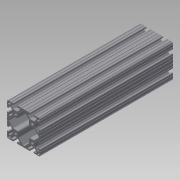
# Autodesk Inventor part: 3030-LITE
Saved by Autodesk Inventor 2013 (Build 170138000, 138)
## iProperties
Created: 2014-04-23
Part Number: 3030-LITE
Material: Generic
Document SubType Name: Modeling
Density: 1 g/cm^3
Vendor: 80/20 Inc.
Engineer: Ross Bowman
Designer: Ross Bowman
Catalog Web Link: 8020.net
Company: 80/20 Inc.
Author: Ross Bowman
Keywords: 80/20 , 8020 , T-Slot , Extrusion
Material: 6105-T5 Aluminum
Autodesk Inventor part; units mm, degrees
ref_plane "YZ Plane" through (0, 0, 0) normal (1, 0, 0) x (0, 1, 0)
ref_plane "XZ Plane" through (0, 0, 0) normal (0, 1, 0) x (-1, 0, 0)
ref_plane "XY Plane" through (0, 0, 0) normal (0, 0, 1) x (1, 0, 0)
sketch "Sketch1" plane through (0, 0, 0) normal (0, 0, 1) x (1, 0, 0)
  circle A0 centre (19.05, -19.05) radius 3.2677
  circle A1 centre (-19.05, -19.05) radius 3.2677
  circle A2 centre (19.05, 19.05) radius 3.2677
  circle A3 centre (-19.05, 19.05) radius 3.2677
  arc A4 (31.2928, -30.9118) -> (30.9118, -31.2928) centre (31.2928, -31.2928) ccw
  line L0 (35.9156, -30.9118) -> (31.2928, -30.9118)
  arc A5 (36.2966, -31.2928) -> (35.9156, -30.9118) centre (35.9156, -31.2928) ccw
  line L1 (36.2966, -33.5026) -> (36.2966, -31.2928)
  arc A6 (33.5026, -36.2966) -> (36.2966, -33.5026) centre (33.5026, -33.5026) ccw
  line L2 (31.2928, -36.2966) -> (33.5026, -36.2966)
  arc A7 (30.9118, -35.9156) -> (31.2928, -36.2966) centre (31.2928, -35.9156) ccw
  line L3 (30.9118, -31.2928) -> (30.9118, -35.9156)
  arc A8 (-35.9156, -30.9118) -> (-36.2966, -31.2928) centre (-35.9156, -31.2928) ccw
  line L4 (-31.2928, -30.9118) -> (-35.9156, -30.9118)
  arc A9 (-30.9118, -31.2928) -> (-31.2928, -30.9118) centre (-31.2928, -31.2928) ccw
  line L5 (-30.9118, -35.9156) -> (-30.9118, -31.2928)
  arc A10 (-31.2928, -36.2966) -> (-30.9118, -35.9156) centre (-31.2928, -35.9156) ccw
  line L6 (-33.5026, -36.2966) -> (-31.2928, -36.2966)
  arc A11 (-36.2966, -33.5026) -> (-33.5026, -36.2966) centre (-33.5026, -33.5026) ccw
  line L7 (-36.2966, -31.2928) -> (-36.2966, -33.5026)
  arc A12 (35.9156, 30.9118) -> (36.2966, 31.2928) centre (35.9156, 31.2928) ccw
  line L8 (31.2928, 30.9118) -> (35.9156, 30.9118)
  arc A13 (30.9118, 31.2928) -> (31.2928, 30.9118) centre (31.2928, 31.2928) ccw
  line L9 (30.9118, 35.9156) -> (30.9118, 31.2928)
  arc A14 (31.2928, 36.2966) -> (30.9118, 35.9156) centre (31.2928, 35.9156) ccw
  line L10 (33.5026, 36.2966) -> (31.2928, 36.2966)
  arc A15 (36.2966, 33.5026) -> (33.5026, 36.2966) centre (33.5026, 33.5026) ccw
  line L11 (36.2966, 31.2928) -> (36.2966, 33.5026)
  arc A16 (-10.9278, 25.0169) -> (-12.319, 21.6583) centre (-7.5692, 21.6583) ccw
  line L12 (-2.0655, 33.8793) -> (-10.9278, 25.0169)
  arc A17 (2.0655, 33.8793) -> (-2.0655, 33.8793) centre (0, 31.8138) ccw
  line L13 (10.9278, 25.0169) -> (2.0655, 33.8793)
  arc A18 (12.319, 21.6583) -> (10.9278, 25.0169) centre (7.5692, 21.6583) ccw
  line L14 (12.319, 15.494) -> (12.319, 21.6583)
  arc A19 (12.319, 15.494) -> (15.494, 12.319) centre (15.494, 15.494) ccw
  line L15 (21.6583, 12.319) -> (15.494, 12.319)
  arc A20 (25.0169, 10.9278) -> (21.6583, 12.319) centre (21.6583, 7.5692) ccw
  line L16 (33.8793, 2.0655) -> (25.0169, 10.9278)
  arc A21 (33.8793, -2.0655) -> (33.8793, 2.0655) centre (31.8138, 0) ccw
  line L17 (25.0169, -10.9278) -> (33.8793, -2.0655)
  arc A22 (21.6583, -12.319) -> (25.0169, -10.9278) centre (21.6583, -7.5692) ccw
  line L18 (15.494, -12.319) -> (21.6583, -12.319)
  arc A23 (15.494, -12.319) -> (12.319, -15.494) centre (15.494, -15.494) ccw
  line L19 (12.319, -21.6583) -> (12.319, -15.494)
  arc A24 (10.9278, -25.0169) -> (12.319, -21.6583) centre (7.5692, -21.6583) ccw
  line L20 (2.0655, -33.8793) -> (10.9278, -25.0169)
  arc A25 (-2.0655, -33.8793) -> (2.0655, -33.8793) centre (0, -31.8138) ccw
  line L21 (-10.9278, -25.0169) -> (-2.0655, -33.8793)
  arc A26 (-12.319, -21.6583) -> (-10.9278, -25.0169) centre (-7.5692, -21.6583) ccw
  line L22 (-12.319, -15.494) -> (-12.319, -21.6583)
  arc A27 (-12.319, -15.494) -> (-15.494, -12.319) centre (-15.494, -15.494) ccw
  line L23 (-21.6583, -12.319) -> (-15.494, -12.319)
  arc A28 (-25.0169, -10.9278) -> (-21.6583, -12.319) centre (-21.6583, -7.5692) ccw
  line L24 (-33.8793, -2.0655) -> (-25.0169, -10.9278)
  arc A29 (-33.8793, 2.0655) -> (-33.8793, -2.0655) centre (-31.8138, 0) ccw
  line L25 (-25.0169, 10.9278) -> (-33.8793, 2.0655)
  arc A30 (-21.6583, 12.319) -> (-25.0169, 10.9278) centre (-21.6583, 7.5692) ccw
  line L26 (-15.494, 12.319) -> (-21.6583, 12.319)
  arc A31 (-15.494, 12.319) -> (-12.319, 15.494) centre (-15.494, 15.494) ccw
  line L27 (-12.319, 21.6583) -> (-12.319, 15.494)
  arc A32 (-31.2928, 30.9118) -> (-30.9118, 31.2928) centre (-31.2928, 31.2928) ccw
  line L28 (-35.9156, 30.9118) -> (-31.2928, 30.9118)
  arc A33 (-36.2966, 31.2928) -> (-35.9156, 30.9118) centre (-35.9156, 31.2928) ccw
  line L29 (-36.2966, 33.5026) -> (-36.2966, 31.2928)
  arc A34 (-33.5026, 36.2966) -> (-36.2966, 33.5026) centre (-33.5026, 33.5026) ccw
  line L30 (-31.2928, 36.2966) -> (-33.5026, 36.2966)
  arc A35 (-30.9118, 35.9156) -> (-31.2928, 36.2966) centre (-31.2928, 35.9156) ccw
  line L31 (-30.9118, 31.2928) -> (-30.9118, 35.9156)
  arc A36 (-3.2004, -38.1) -> (-4.7244, -38.1) centre (-3.9624, -38.1) ccw
  line L32 (-3.2004, -38.1) -> (3.2004, -38.1)
  arc A37 (4.7244, -38.1) -> (3.2004, -38.1) centre (3.9624, -38.1) ccw
  line L33 (4.7244, -38.1) -> (9.5504, -38.1)
  arc A38 (11.0744, -38.1) -> (9.5504, -38.1) centre (10.3124, -38.1) ccw
  line L34 (11.0744, -38.1) -> (13.4107, -38.1)
  arc A39 (13.4107, -38.1) -> (14.986, -36.5252) centre (13.4112, -36.5252) ccw
  line L35 (14.986, -36.5252) -> (14.986, -35.6108)
  arc A40 (14.986, -35.6108) -> (13.4112, -34.036) centre (13.4112, -35.6108) ccw
  line L36 (13.4112, -34.036) -> (12.5733, -34.036)
  arc A41 (12.5733, -34.036) -> (12.192, -34.417) centre (12.573, -34.417) ccw
  line L37 (12.192, -34.417) -> (12.192, -34.4932)
  arc A42 (11.811, -34.8742) -> (12.192, -34.4932) centre (11.811, -34.4932) ccw
  line L38 (11.811, -34.8742) -> (10.033, -34.8742)
  arc A43 (8.763, -33.6042) -> (10.033, -34.8742) centre (10.033, -33.6042) ccw
  line L39 (8.763, -33.6042) -> (8.763, -32.0193)
  arc A44 (9.135, -31.1203) -> (8.763, -32.0193) centre (10.033, -32.0183) ccw
  line L40 (9.135, -31.1203) -> (13.0807, -27.1745)
  arc A45 (16.4417, -25.781) -> (13.0807, -27.1745) centre (16.4417, -30.5308) ccw
  line L41 (16.4417, -25.781) -> (21.6583, -25.781)
  arc A46 (25.0169, -27.1722) -> (21.6583, -25.781) centre (21.6583, -30.5308) ccw
  line L42 (25.0169, -27.1722) -> (28.965, -31.1203)
  arc A47 (29.337, -32.0183) -> (28.965, -31.1203) centre (28.067, -32.0183) ccw
  line L43 (29.337, -32.0183) -> (29.337, -33.6018)
  arc A48 (28.067, -34.8742) -> (29.337, -33.6018) centre (28.067, -33.6042) ccw
  line L44 (28.067, -34.8742) -> (26.289, -34.8742)
  arc A49 (25.908, -34.4932) -> (26.289, -34.8742) centre (26.289, -34.4932) ccw
  line L45 (25.908, -34.4932) -> (25.908, -34.417)
  arc A50 (25.908, -34.417) -> (25.527, -34.036) centre (25.527, -34.417) ccw
  line L46 (25.527, -34.036) -> (24.6894, -34.036)
  arc A51 (24.6894, -34.036) -> (23.114, -35.6108) centre (24.6888, -35.6108) ccw
  line L47 (23.114, -35.6108) -> (23.114, -36.5252)
  arc A52 (23.114, -36.5252) -> (24.6888, -38.1) centre (24.6888, -36.5252) ccw
  line L48 (24.6888, -38.1) -> (27.0256, -38.1)
  arc A53 (28.5496, -38.1) -> (27.0256, -38.1) centre (27.7876, -38.1) ccw
  line L49 (28.5496, -38.1) -> (33.3756, -38.1)
  arc A54 (34.8996, -38.0999) -> (33.3756, -38.1) centre (34.1376, -38.1) ccw
  arc A55 (34.8996, -38.0999) -> (38.0999, -34.8996) centre (34.925, -34.925) ccw
  arc A56 (38.1, -33.3756) -> (38.0999, -34.8996) centre (38.1, -34.1376) ccw
  line L50 (38.1, -33.3756) -> (38.1, -28.5496)
  arc A57 (38.1, -27.0256) -> (38.1, -28.5496) centre (38.1, -27.7876) ccw
  line L51 (38.1, -27.0256) -> (38.1, -24.6893)
  arc A58 (38.1, -24.6893) -> (36.5252, -23.114) centre (36.5252, -24.6888) ccw
  line L52 (36.5252, -23.114) -> (35.6118, -23.114)
  arc A59 (35.6118, -23.114) -> (34.036, -24.6888) centre (35.6108, -24.6888) ccw
  line L53 (34.036, -24.6888) -> (34.036, -25.5253)
  arc A60 (34.036, -25.5253) -> (34.417, -25.908) centre (34.417, -25.527) ccw
  line L54 (34.417, -25.908) -> (34.4929, -25.908)
  arc A61 (34.8742, -26.289) -> (34.4929, -25.908) centre (34.4932, -26.289) ccw
  line L55 (34.8742, -26.289) -> (34.8742, -28.067)
  arc A62 (33.6042, -29.337) -> (34.8742, -28.067) centre (33.6042, -28.067) ccw
  line L56 (33.6042, -29.337) -> (32.0183, -29.337)
  arc A63 (31.1203, -28.965) -> (32.0183, -29.337) centre (32.0183, -28.067) ccw
  line L57 (31.1203, -28.965) -> (27.1749, -25.0196)
  arc A64 (25.781, -21.6583) -> (27.1749, -25.0196) centre (30.5308, -21.6583) ccw
  line L58 (25.781, -21.6583) -> (25.781, -16.4417)
  arc A65 (27.1722, -13.0831) -> (25.781, -16.4417) centre (30.5308, -16.4417) ccw
  line L59 (27.1722, -13.0831) -> (31.1203, -9.135)
  arc A66 (32.0183, -8.763) -> (31.1203, -9.135) centre (32.0183, -10.033) ccw
  line L60 (32.0183, -8.763) -> (33.6042, -8.763)
  arc A67 (34.8742, -10.033) -> (33.6042, -8.763) centre (33.6042, -10.033) ccw
  line L61 (34.8742, -10.033) -> (34.8742, -11.811)
  arc A68 (34.4932, -12.192) -> (34.8742, -11.811) centre (34.4932, -11.811) ccw
  line L62 (34.4932, -12.192) -> (34.4171, -12.192)
  arc A69 (34.4171, -12.192) -> (34.036, -12.573) centre (34.417, -12.573) ccw
  line L63 (34.036, -12.573) -> (34.036, -13.4078)
  arc A70 (34.036, -13.4078) -> (35.6108, -14.986) centre (35.6108, -13.4112) ccw
  line L64 (35.6108, -14.986) -> (36.5242, -14.986)
  arc A71 (36.5242, -14.986) -> (38.1, -13.4112) centre (36.5252, -13.4112) ccw
  line L65 (38.1, -13.4112) -> (38.1, -11.0744)
  arc A72 (38.1, -9.5504) -> (38.1, -11.0744) centre (38.1, -10.3124) ccw
  line L66 (38.1, -9.5504) -> (38.1, -4.7244)
  arc A73 (38.1, -3.2004) -> (38.1, -4.7244) centre (38.1, -3.9624) ccw
  line L67 (38.1, -3.2004) -> (38.1, 3.2004)
  arc A74 (38.1, 4.7244) -> (38.1, 3.2004) centre (38.1, 3.9624) ccw
  line L68 (38.1, 4.7244) -> (38.1, 9.5504)
  arc A75 (38.1, 11.0744) -> (38.1, 9.5504) centre (38.1, 10.3124) ccw
  line L69 (38.1, 11.0744) -> (38.1, 13.4107)
  arc A76 (38.1, 13.4107) -> (36.5252, 14.986) centre (36.5252, 13.4112) ccw
  line L70 (36.5252, 14.986) -> (35.6113, 14.986)
  arc A77 (35.6113, 14.986) -> (34.036, 13.4112) centre (35.6108, 13.4112) ccw
  line L71 (34.036, 13.4112) -> (34.036, 12.5732)
  arc A78 (34.036, 12.5732) -> (34.417, 12.192) centre (34.417, 12.573) ccw
  line L72 (34.417, 12.192) -> (34.493, 12.192)
  arc A79 (34.8742, 11.811) -> (34.493, 12.192) centre (34.4932, 11.811) ccw
  line L73 (34.8742, 11.811) -> (34.8742, 10.033)
  arc A80 (33.6042, 8.763) -> (34.8742, 10.033) centre (33.6042, 10.033) ccw
  line L74 (33.6042, 8.763) -> (32.0183, 8.763)
  arc A81 (31.1203, 9.135) -> (32.0183, 8.763) centre (32.0183, 10.033) ccw
  line L75 (31.1203, 9.135) -> (27.173, 13.0823)
  arc A82 (25.781, 16.4417) -> (27.173, 13.0823) centre (30.5308, 16.4417) ccw
  line L76 (25.781, 16.4417) -> (25.781, 21.6572)
  arc A83 (27.1722, 25.0169) -> (25.781, 21.6572) centre (30.5308, 21.6583) ccw
  line L77 (27.1722, 25.0169) -> (31.1203, 28.965)
  arc A84 (32.0183, 29.337) -> (31.1203, 28.965) centre (32.0183, 28.067) ccw
  line L78 (32.0183, 29.337) -> (33.6042, 29.337)
  arc A85 (34.8742, 28.067) -> (33.6042, 29.337) centre (33.6042, 28.067) ccw
  line L79 (34.8742, 28.067) -> (34.8742, 26.2892)
  arc A86 (34.4932, 25.908) -> (34.8742, 26.2892) centre (34.4932, 26.289) ccw
  line L80 (34.4932, 25.908) -> (34.4172, 25.908)
  arc A87 (34.4172, 25.908) -> (34.036, 25.527) centre (34.417, 25.527) ccw
  line L81 (34.036, 25.527) -> (34.036, 24.6893)
  arc A88 (34.036, 24.6893) -> (35.6108, 23.114) centre (35.6108, 24.6888) ccw
  line L82 (35.6108, 23.114) -> (36.5247, 23.114)
  arc A89 (36.5247, 23.114) -> (38.1, 24.6888) centre (36.5252, 24.6888) ccw
  line L83 (38.1, 24.6888) -> (38.1, 27.0256)
  arc A90 (38.1, 28.5496) -> (38.1, 27.0256) centre (38.1, 27.7876) ccw
  line L84 (38.1, 28.5496) -> (38.1, 33.3756)
  arc A91 (38.0999, 34.8996) -> (38.1, 33.3756) centre (38.1, 34.1376) ccw
  arc A92 (38.0999, 34.8996) -> (34.8996, 38.0999) centre (34.925, 34.925) ccw
  arc A93 (33.3756, 38.1) -> (34.8996, 38.0999) centre (34.1376, 38.1) ccw
  line L85 (33.3756, 38.1) -> (28.5496, 38.1)
  arc A94 (27.0256, 38.1) -> (28.5496, 38.1) centre (27.7876, 38.1) ccw
  line L86 (27.0256, 38.1) -> (24.6893, 38.1)
  arc A95 (24.6893, 38.1) -> (23.114, 36.5252) centre (24.6888, 36.5252) ccw
  line L87 (23.114, 36.5252) -> (23.114, 35.6113)
  arc A96 (23.114, 35.6113) -> (24.6888, 34.036) centre (24.6888, 35.6108) ccw
  line L88 (24.6888, 34.036) -> (25.527, 34.036)
  arc A97 (25.527, 34.036) -> (25.908, 34.417) centre (25.527, 34.417) ccw
  line L89 (25.908, 34.417) -> (25.908, 34.4932)
  arc A98 (26.289, 34.8742) -> (25.908, 34.4932) centre (26.289, 34.4932) ccw
  line L90 (26.289, 34.8742) -> (28.067, 34.8742)
  arc A99 (29.337, 33.6042) -> (28.067, 34.8742) centre (28.067, 33.6042) ccw
  line L91 (29.337, 33.6042) -> (29.337, 32.0183)
  arc A100 (28.965, 31.1203) -> (29.337, 32.0183) centre (28.067, 32.0183) ccw
  line L92 (28.965, 31.1203) -> (25.0177, 27.173)
  arc A101 (21.6583, 25.781) -> (25.0177, 27.173) centre (21.6583, 30.5308) ccw
  line L93 (21.6583, 25.781) -> (16.4428, 25.781)
  arc A102 (13.0831, 27.1722) -> (16.4428, 25.781) centre (16.4417, 30.5308) ccw
  line L94 (13.0831, 27.1722) -> (9.135, 31.1203)
  arc A103 (8.763, 32.0183) -> (9.135, 31.1203) centre (10.033, 32.0183) ccw
  line L95 (8.763, 32.0183) -> (8.763, 33.6042)
  arc A104 (10.033, 34.8742) -> (8.763, 33.6042) centre (10.033, 33.6042) ccw
  line L96 (10.033, 34.8742) -> (11.8108, 34.8742)
  arc A105 (12.192, 34.4932) -> (11.8108, 34.8742) centre (11.811, 34.4932) ccw
  line L97 (12.192, 34.4932) -> (12.192, 34.417)
  arc A106 (12.192, 34.417) -> (12.573, 34.036) centre (12.573, 34.417) ccw
  line L98 (12.573, 34.036) -> (13.4107, 34.036)
  arc A107 (13.4107, 34.036) -> (14.986, 35.6108) centre (13.4112, 35.6108) ccw
  line L99 (14.986, 35.6108) -> (14.986, 36.5247)
  arc A108 (14.986, 36.5247) -> (13.4112, 38.1) centre (13.4112, 36.5252) ccw
  line L100 (13.4112, 38.1) -> (11.0744, 38.1)
  arc A109 (9.5504, 38.1) -> (11.0744, 38.1) centre (10.3124, 38.1) ccw
  line L101 (9.5504, 38.1) -> (4.7244, 38.1)
  arc A110 (3.2004, 38.1) -> (4.7244, 38.1) centre (3.9624, 38.1) ccw
  line L102 (3.2004, 38.1) -> (-3.2004, 38.1)
  arc A111 (-4.7244, 38.1) -> (-3.2004, 38.1) centre (-3.9624, 38.1) ccw
  line L103 (-4.7244, 38.1) -> (-9.5504, 38.1)
  arc A112 (-11.0744, 38.1) -> (-9.5504, 38.1) centre (-10.3124, 38.1) ccw
  line L104 (-11.0744, 38.1) -> (-13.4107, 38.1)
  arc A113 (-13.4107, 38.1) -> (-14.986, 36.5252) centre (-13.4112, 36.5252) ccw
  line L105 (-14.986, 36.5252) -> (-14.986, 35.6108)
  arc A114 (-14.986, 35.6108) -> (-13.4112, 34.036) centre (-13.4112, 35.6108) ccw
  line L106 (-13.4112, 34.036) -> (-12.5733, 34.036)
  arc A115 (-12.5733, 34.036) -> (-12.192, 34.417) centre (-12.573, 34.417) ccw
  line L107 (-12.192, 34.417) -> (-12.192, 34.4932)
  arc A116 (-11.811, 34.8742) -> (-12.192, 34.4932) centre (-11.811, 34.4932) ccw
  line L108 (-11.811, 34.8742) -> (-10.033, 34.8742)
  arc A117 (-8.763, 33.6042) -> (-10.033, 34.8742) centre (-10.033, 33.6042) ccw
  line L109 (-8.763, 33.6042) -> (-8.763, 32.0194)
  arc A118 (-9.135, 31.1203) -> (-8.763, 32.0194) centre (-10.033, 32.0183) ccw
  line L110 (-9.135, 31.1203) -> (-13.0807, 27.1746)
  arc A119 (-16.4417, 25.781) -> (-13.0807, 27.1746) centre (-16.4417, 30.5308) ccw
  line L111 (-16.4417, 25.781) -> (-21.6583, 25.781)
  arc A120 (-25.0169, 27.1722) -> (-21.6583, 25.781) centre (-21.6583, 30.5308) ccw
  line L112 (-25.0169, 27.1722) -> (-28.965, 31.1203)
  arc A121 (-29.337, 32.0183) -> (-28.965, 31.1203) centre (-28.067, 32.0183) ccw
  line L113 (-29.337, 32.0183) -> (-29.337, 33.6018)
  arc A122 (-28.067, 34.8742) -> (-29.337, 33.6018) centre (-28.067, 33.6042) ccw
  line L114 (-28.067, 34.8742) -> (-26.289, 34.8742)
  arc A123 (-25.908, 34.4932) -> (-26.289, 34.8742) centre (-26.289, 34.4932) ccw
  line L115 (-25.908, 34.4932) -> (-25.908, 34.417)
  arc A124 (-25.908, 34.417) -> (-25.527, 34.036) centre (-25.527, 34.417) ccw
  line L116 (-25.527, 34.036) -> (-24.6894, 34.036)
  arc A125 (-24.6894, 34.036) -> (-23.114, 35.6108) centre (-24.6888, 35.6108) ccw
  line L117 (-23.114, 35.6108) -> (-23.114, 36.5252)
  arc A126 (-23.114, 36.5252) -> (-24.6888, 38.1) centre (-24.6888, 36.5252) ccw
  line L118 (-24.6888, 38.1) -> (-27.0256, 38.1)
  arc A127 (-28.5496, 38.1) -> (-27.0256, 38.1) centre (-27.7876, 38.1) ccw
  line L119 (-28.5496, 38.1) -> (-33.3756, 38.1)
  arc A128 (-34.8996, 38.0999) -> (-33.3756, 38.1) centre (-34.1376, 38.1) ccw
  arc A129 (-34.8996, 38.0999) -> (-38.0999, 34.8996) centre (-34.925, 34.925) ccw
  arc A130 (-38.1, 33.3756) -> (-38.0999, 34.8996) centre (-38.1, 34.1376) ccw
  line L120 (-38.1, 33.3756) -> (-38.1, 28.5496)
  arc A131 (-38.1, 27.0256) -> (-38.1, 28.5496) centre (-38.1, 27.7876) ccw
  line L121 (-38.1, 27.0256) -> (-38.1, 24.6893)
  arc A132 (-38.1, 24.6893) -> (-36.5252, 23.114) centre (-36.5252, 24.6888) ccw
  line L122 (-36.5252, 23.114) -> (-35.6118, 23.114)
  arc A133 (-35.6118, 23.114) -> (-34.036, 24.6888) centre (-35.6108, 24.6888) ccw
  line L123 (-34.036, 24.6888) -> (-34.036, 25.5253)
  arc A134 (-34.036, 25.5253) -> (-34.417, 25.908) centre (-34.417, 25.527) ccw
  line L124 (-34.417, 25.908) -> (-34.4929, 25.908)
  arc A135 (-34.8742, 26.289) -> (-34.4929, 25.908) centre (-34.4932, 26.289) ccw
  line L125 (-34.8742, 26.289) -> (-34.8742, 28.067)
  arc A136 (-33.6042, 29.337) -> (-34.8742, 28.067) centre (-33.6042, 28.067) ccw
  line L126 (-33.6042, 29.337) -> (-32.0183, 29.337)
  arc A137 (-31.1203, 28.965) -> (-32.0183, 29.337) centre (-32.0183, 28.067) ccw
  line L127 (-31.1203, 28.965) -> (-27.1749, 25.0196)
  arc A138 (-25.781, 21.6583) -> (-27.1749, 25.0196) centre (-30.5308, 21.6583) ccw
  line L128 (-25.781, 21.6583) -> (-25.781, 16.4417)
  arc A139 (-27.1722, 13.0831) -> (-25.781, 16.4417) centre (-30.5308, 16.4417) ccw
  line L129 (-27.1722, 13.0831) -> (-31.1203, 9.135)
  arc A140 (-32.0183, 8.763) -> (-31.1203, 9.135) centre (-32.0183, 10.033) ccw
  line L130 (-32.0183, 8.763) -> (-33.6042, 8.763)
  arc A141 (-34.8742, 10.033) -> (-33.6042, 8.763) centre (-33.6042, 10.033) ccw
  line L131 (-34.8742, 10.033) -> (-34.8742, 11.811)
  arc A142 (-34.4932, 12.192) -> (-34.8742, 11.811) centre (-34.4932, 11.811) ccw
  line L132 (-34.4932, 12.192) -> (-34.4171, 12.192)
  arc A143 (-34.4171, 12.192) -> (-34.036, 12.573) centre (-34.417, 12.573) ccw
  line L133 (-34.036, 12.573) -> (-34.036, 13.4078)
  arc A144 (-34.036, 13.4078) -> (-35.6108, 14.986) centre (-35.6108, 13.4112) ccw
  line L134 (-35.6108, 14.986) -> (-36.5242, 14.986)
  arc A145 (-36.5242, 14.986) -> (-38.1, 13.4112) centre (-36.5252, 13.4112) ccw
  line L135 (-38.1, 13.4112) -> (-38.1, 11.0744)
  arc A146 (-38.1, 9.5504) -> (-38.1, 11.0744) centre (-38.1, 10.3124) ccw
  line L136 (-38.1, 9.5504) -> (-38.1, 4.7244)
  arc A147 (-38.1, 3.2004) -> (-38.1, 4.7244) centre (-38.1, 3.9624) ccw
  line L137 (-38.1, 3.2004) -> (-38.1, -3.2004)
  arc A148 (-38.1, -4.7244) -> (-38.1, -3.2004) centre (-38.1, -3.9624) ccw
  line L138 (-38.1, -4.7244) -> (-38.1, -9.5504)
  arc A149 (-38.1, -11.0744) -> (-38.1, -9.5504) centre (-38.1, -10.3124) ccw
  line L139 (-38.1, -11.0744) -> (-38.1, -13.4107)
  arc A150 (-38.1, -13.4107) -> (-36.5252, -14.986) centre (-36.5252, -13.4112) ccw
  line L140 (-36.5252, -14.986) -> (-35.6113, -14.986)
  arc A151 (-35.6113, -14.986) -> (-34.036, -13.4112) centre (-35.6108, -13.4112) ccw
  line L141 (-34.036, -13.4112) -> (-34.036, -12.5732)
  arc A152 (-34.036, -12.5732) -> (-34.417, -12.192) centre (-34.417, -12.573) ccw
  line L142 (-34.417, -12.192) -> (-34.493, -12.192)
  arc A153 (-34.8742, -11.811) -> (-34.493, -12.192) centre (-34.4932, -11.811) ccw
  line L143 (-34.8742, -11.811) -> (-34.8742, -10.033)
  arc A154 (-33.6042, -8.763) -> (-34.8742, -10.033) centre (-33.6042, -10.033) ccw
  line L144 (-33.6042, -8.763) -> (-32.0183, -8.763)
  arc A155 (-31.1203, -9.135) -> (-32.0183, -8.763) centre (-32.0183, -10.033) ccw
  line L145 (-31.1203, -9.135) -> (-27.173, -13.0823)
  arc A156 (-25.781, -16.4417) -> (-27.173, -13.0823) centre (-30.5308, -16.4417) ccw
  line L146 (-25.781, -16.4417) -> (-25.781, -21.6572)
  arc A157 (-27.1722, -25.0169) -> (-25.781, -21.6572) centre (-30.5308, -21.6583) ccw
  line L147 (-27.1722, -25.0169) -> (-31.1203, -28.965)
  arc A158 (-32.0183, -29.337) -> (-31.1203, -28.965) centre (-32.0183, -28.067) ccw
  line L148 (-32.0183, -29.337) -> (-33.6042, -29.337)
  arc A159 (-34.8742, -28.067) -> (-33.6042, -29.337) centre (-33.6042, -28.067) ccw
  line L149 (-34.8742, -28.067) -> (-34.8742, -26.2892)
  arc A160 (-34.4932, -25.908) -> (-34.8742, -26.2892) centre (-34.4932, -26.289) ccw
  line L150 (-34.4932, -25.908) -> (-34.4172, -25.908)
  arc A161 (-34.4172, -25.908) -> (-34.036, -25.527) centre (-34.417, -25.527) ccw
  line L151 (-34.036, -25.527) -> (-34.036, -24.6893)
  arc A162 (-34.036, -24.6893) -> (-35.6108, -23.114) centre (-35.6108, -24.6888) ccw
  line L152 (-35.6108, -23.114) -> (-36.5247, -23.114)
  arc A163 (-36.5247, -23.114) -> (-38.1, -24.6888) centre (-36.5252, -24.6888) ccw
  line L153 (-38.1, -24.6888) -> (-38.1, -27.0256)
  arc A164 (-38.1, -28.5496) -> (-38.1, -27.0256) centre (-38.1, -27.7876) ccw
  line L154 (-38.1, -28.5496) -> (-38.1, -33.3756)
  arc A165 (-38.0999, -34.8996) -> (-38.1, -33.3756) centre (-38.1, -34.1376) ccw
  arc A166 (-38.0999, -34.8996) -> (-34.8996, -38.0999) centre (-34.925, -34.925) ccw
  arc A167 (-33.3756, -38.1) -> (-34.8996, -38.0999) centre (-34.1376, -38.1) ccw
  line L155 (-33.3756, -38.1) -> (-28.5496, -38.1)
  arc A168 (-27.0256, -38.1) -> (-28.5496, -38.1) centre (-27.7876, -38.1) ccw
  line L156 (-27.0256, -38.1) -> (-24.6893, -38.1)
  arc A169 (-24.6893, -38.1) -> (-23.114, -36.5252) centre (-24.6888, -36.5252) ccw
  line L157 (-23.114, -36.5252) -> (-23.114, -35.6113)
  arc A170 (-23.114, -35.6113) -> (-24.6888, -34.036) centre (-24.6888, -35.6108) ccw
  line L158 (-24.6888, -34.036) -> (-25.527, -34.036)
  arc A171 (-25.527, -34.036) -> (-25.908, -34.417) centre (-25.527, -34.417) ccw
  line L159 (-25.908, -34.417) -> (-25.908, -34.4932)
  arc A172 (-26.289, -34.8742) -> (-25.908, -34.4932) centre (-26.289, -34.4932) ccw
  line L160 (-26.289, -34.8742) -> (-28.067, -34.8742)
  arc A173 (-29.337, -33.6042) -> (-28.067, -34.8742) centre (-28.067, -33.6042) ccw
  line L161 (-29.337, -33.6042) -> (-29.337, -32.0183)
  arc A174 (-28.965, -31.1203) -> (-29.337, -32.0183) centre (-28.067, -32.0183) ccw
  line L162 (-28.965, -31.1203) -> (-25.0177, -27.173)
  arc A175 (-21.6583, -25.781) -> (-25.0177, -27.173) centre (-21.6583, -30.5308) ccw
  line L163 (-21.6583, -25.781) -> (-16.4428, -25.781)
  arc A176 (-13.0831, -27.1722) -> (-16.4428, -25.781) centre (-16.4417, -30.5308) ccw
  line L164 (-13.0831, -27.1722) -> (-9.135, -31.1203)
  arc A177 (-8.763, -32.0183) -> (-9.135, -31.1203) centre (-10.033, -32.0183) ccw
  line L165 (-8.763, -32.0183) -> (-8.763, -33.6042)
  arc A178 (-10.033, -34.8742) -> (-8.763, -33.6042) centre (-10.033, -33.6042) ccw
  line L166 (-10.033, -34.8742) -> (-11.8108, -34.8742)
  arc A179 (-12.192, -34.4932) -> (-11.8108, -34.8742) centre (-11.811, -34.4932) ccw
  line L167 (-12.192, -34.4932) -> (-12.192, -34.417)
  arc A180 (-12.192, -34.417) -> (-12.573, -34.036) centre (-12.573, -34.417) ccw
  line L168 (-12.573, -34.036) -> (-13.4107, -34.036)
  arc A181 (-13.4107, -34.036) -> (-14.986, -35.6108) centre (-13.4112, -35.6108) ccw
  line L169 (-14.986, -35.6108) -> (-14.986, -36.5247)
  arc A182 (-14.986, -36.5247) -> (-13.4112, -38.1) centre (-13.4112, -36.5252) ccw
  line L170 (-13.4112, -38.1) -> (-11.0744, -38.1)
  arc A183 (-9.5504, -38.1) -> (-11.0744, -38.1) centre (-10.3124, -38.1) ccw
  line L171 (-9.5504, -38.1) -> (-4.7244, -38.1)
  point P0 (0, 0)
  constraints: 360 point on circle, 344 end point, 184 centre point
extrude "Extrusion1" add sketch "Sketch1" against normal blind 304.8
body "Solid1"
